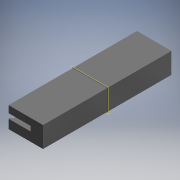
# Autodesk Inventor part: cord holder
Saved by Autodesk Inventor 2019 (Build 230136000, 136)
## iProperties
Part Number: cord holder
Material: Generic
Document SubType Name: Modeling
Designer: Delta
Appearance: Default
Author: Delta
Autodesk Inventor part; units mm, degrees
ref_plane "YZ Plane" through (0, 0, 0) normal (1, 0, 0) x (0, 1, 0)
ref_plane "XZ Plane" through (0, 0, 0) normal (0, 1, 0) x (-1, 0, 0)
ref_plane "XY Plane" through (0, 0, 0) normal (0, 0, 1) x (1, 0, 0)
sketch "Sketch1" plane through (0, 0, 0) normal (0, 1, 0) x (-1, 0, 0)
  line L0 (0, 0) -> (6.35, 0)
  line L1 (6.35, 0) -> (6.35, -27.94)
  line L2 (6.35, -27.94) -> (0, -27.94)
  line L3 (0, -27.94) -> (0, 0)
  dimension "d0" = 6.35
  dimension "d1" = 27.94
  constraints: 8 end point, 3 perpendicular, 1 horizontal
  measures "d0" distance of L0.start L0.end
  measures "d1" distance of L0.end L1.end
extrude "Extrusion1" add sketch "Sketch1" along normal blind 1.5875
sketch "Sketch2" plane through (-6.35, 0, 0) normal (0, 0, 1) x (1, 0, 0)
  line L0 (0, 1.5875) -> (6.35, 1.5875) projected
  line L1 (6.35, 1.5875) -> (6.35, 3.175)
  line L2 (6.35, 3.175) -> (5.08, 3.175)
  line L3 (5.08, 3.175) -> (5.08, 1.5875)
  line L4 (0, 1.5875) -> (6.35, 1.5875)
  line L5 (6.35, 1.5875) -> (6.35, 0)
  line L6 (6.35, 0) -> (0, 0)
  line L7 (0, 0) -> (0, 1.5875)
  point P0 (1.27, 1.5875)
  dimension "d4" = 1.27
  dimension "d7" = 1.5875
  constraints: 14 end point, 2 parallel, 2 perpendicular, 2 point on line, 1 horizontal
  measures "d4" distance of L1.end L2.end
  measures "d7" distance between parallel lines of L0 L2
ref_plane "Work Plane2" through (0, 1.5875, 0) normal (1, 0, 0) x (0, 0, -1)
sketch "Sketch3" plane through (0, 1.5875, 0) normal (1, 0, 0) x (0, 0, -1)
  line L0 (0, 0) -> (27.94, 0) projected
  line L1 (27.94, -1.5875) -> (0, -1.5875) projected
  line L2 (27.94, -1.5875) -> (27.94, 0) projected
  line L3 (27.94, -1.5875) -> (-1.5875, -1.5875) projected
  line L4 (27.94, -1.5875) -> (-1.5875, -1.5875)
  line L5 (-1.5875, -1.5875) -> (-1.5875, 3.175)
  line L6 (-1.5875, 3.175) -> (27.94, 3.175)
  line L7 (27.94, 3.175) -> (27.94, -1.5875)
  line L8 (0, -1.5875) -> (0, 0) projected
  constraints: 8 end point, 2 parallel, 1 horizontal, 1 perpendicular
extrude "Extrusion3" add sketch "Sketch3" along normal blind 1.5875
ref_plane "Work Plane3" through (0, 1.5875, 0) normal (-1, 0, 0) x (0, 0, 1)
sketch "Sketch4" plane through (0, 1.5875, 0) normal (-1, 0, 0) x (0, 0, 1)
  line L0 (1.5875, 0) -> (1.5875, 1.5875) projected
  line L1 (1.5875, 1.5875) -> (1.5875, 2.3812)
  line L2 (1.5875, 3.175) -> (1.5875, -1.5875) projected
  line L3 (-27.94, 3.175) -> (1.5875, 3.175) projected
  line L4 (0, 1.5875) -> (1.5875, 1.5875) projected
  line L5 (1.5875, 3.175) -> (1.5875, 1.5875)
  line L6 (-27.94, 0) -> (-27.94, 3.175) projected
  line L7 (1.5875, 1.5875) -> (-27.94, 1.5875)
  line L8 (-27.94, 1.5875) -> (-27.94, 3.175)
  line L9 (-27.94, 3.175) -> (1.5875, 3.175)
  point P0 (0, -1.5875)
  constraints: 10 end point, 2 perpendicular, 1 collinear, 1 point on line, 1 vertical
extrude "Extrusion4" add sketch "Sketch4" along normal up to surface (6.35 mm away)
extrude "Extrusion5" add sketch "Sketch2" along normal blind 1.5875
ref_plane "Work Plane4" through (-6.35, 0, -13.1763) normal (0, 0, -1) x (-1, 0, 0)
mirror "Mirror2" about plane through (-6.35, 0, -13.1763) normal (0, 0, -1) of "Extrusion5"
sketch "Sketch5" plane through (-6.35, 0, -27.94) normal (0, 0, -1) x (-1, 0, 0)
  line L0 (0, 1.5875) -> (0, 0) projected
  line L1 (0, 1.5875) -> (0, 2.0585)
  line L2 (0, 2.0585) -> (-5.08, 2.0585)
  line L3 (-5.08, 3.175) -> (-5.08, 1.5875) projected
  line L4 (-5.08, 1.5875) -> (0, 1.5875) projected
  line L5 (-5.08, 1.5875) -> (0, 1.5875)
  point P0 (-6.35, 0)
  constraints: 6 end point, 1 collinear, 1 perpendicular, 1 point on line, 1 vertical
extrude "Extrusion6" add sketch "Sketch5" against normal blind 0.5292
mirror "Mirror3" about plane through (-6.35, 0, -13.1763) normal (0, 0, -1) of "Extrusion6"
body "Solid1"
